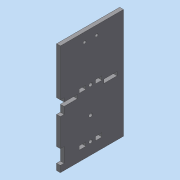
# Autodesk Inventor part: X-Motor-Housing_Side
Saved by Autodesk Inventor 2016 SP1 (Build 200210100, 210)
## iProperties
Created: 2016-02-23
Part Number: X-Motor-Housing_Side
Material: Generic
Document SubType Name: Modeling
Designer: Mohamed A.
Density: 1 g/cm^3
Appearance: Default
Author: Mohamed A.
Autodesk Inventor part; units mm, degrees
ref_plane "YZ Plane" through (0, 0, 0) normal (1, 0, 0) x (0, 1, 0)
ref_plane "XZ Plane" through (0, 0, 0) normal (0, 1, 0) x (-1, 0, 0)
ref_plane "XY Plane" through (0, 0, 0) normal (0, 0, 1) x (1, 0, 0)
sketch "Sketch2" plane through (0, 0, 0) normal (1, 0, 0) x (0, 1, 0)
  line L0 (-21, 22.5) -> (-21, 19.5)
  line L1 (-21, -11) -> (-21, -27.5)
  line L2 (-21, -27.5) -> (26, -27.5)
  line L3 (26, -27.5) -> (26, 27.5)
  line L4 (26, 27.5) -> (-21, 27.5)
  line L5 (-21, 27.5) -> (-21, 22.5)
  line L6 (26, 27.5) -> (26, 57.5)
  line L7 (26, 57.5) -> (-21, 57.5)
  line L8 (-21, 57.5) -> (-21, 27.5)
  circle A0 centre (4.7625, 50.5) radius 1.15
  circle A1 centre (-4.7625, 50.5) radius 1.15
  line L9 (4.7625, 50.5) -> (0, 50.5) construction
  line L10 (0, 50.5) -> (-4.7625, 50.5) construction
  line L11 (-21, 22.5) -> (-24, 22.5)
  line L12 (-24, 22.5) -> (-24, 57.5)
  line L13 (-24, 57.5) -> (-21, 57.5)
  line L14 (-21, -22.5) -> (-24, -22.5)
  line L15 (-24, -22.5) -> (-24, -27.5)
  line L16 (-24, -27.5) -> (-21, -27.5)
  line L17 (-21, -11) -> (-24, -11)
  line L18 (-24, -11) -> (-24, 11)
  line L19 (-24, 11) -> (-21, 11)
  line L20 (-21, 11) -> (-21, -11)
  line L21 (-21, 16.5) -> (-21, 11)
  line L22 (-21, 19.5) -> (-21, 16.5)
  circle A2 centre (0, 0) radius 1.4
  line L23 (10.5, 19.5) -> (21, 19.5) projected
  line L24 (10.5, 19.5) -> (10.5, 16.5) projected
  line L25 (21, 16.5) -> (10.5, 16.5) projected
  line L26 (21, 19.5) -> (21, 16.5) projected
  line L27 (3.75, 19.5) -> (9, 19.5) projected
  line L28 (9, 19.5) -> (9, 22.5) projected
  line L29 (3.75, 22.5) -> (9, 22.5) projected
  line L30 (3.75, 19.5) -> (3.75, 22.5) projected
  line L31 (-9, 19.5) -> (-3.75, 19.5) projected
  line L32 (-3.75, 19.5) -> (-3.75, 22.5) projected
  line L33 (-9, 22.5) -> (-3.75, 22.5) projected
  line L34 (-9, 19.5) -> (-9, 22.5) projected
  line L35 (-24, 19.5) -> (-10.5, 19.5) projected
  line L36 (-24, 19.5) -> (-24, 16.5) projected
  line L37 (-10.5, 16.5) -> (-24, 16.5) projected
  line L38 (-10.5, 19.5) -> (-10.5, 16.5) projected
  line L39 (0, -44.5) -> (0, 74.5) construction
  line L40 (-34, 0) -> (36, 0) construction
  line L41 (3.75, 22.5) -> (-3.75, 19.5) construction
  line L42 (3.75, 19.5) -> (-3.75, 22.5) construction
  circle A3 centre (0, 21) radius 1.4
  line L43 (-10.5, 16.5) -> (-21, 16.5)
  line L44 (-10.5, 16.5) -> (-10.5, 19.5)
  line L45 (-10.5, 19.5) -> (-21, 19.5)
  line L46 (-21, 16.5) -> (-21, 19.5)
  line L47 (9, -16.5) -> (3.75, -16.5) projected
  line L48 (3.75, -16.5) -> (3.75, -19.5) projected
  line L49 (9, -19.5) -> (3.75, -19.5) projected
  line L50 (9, -16.5) -> (9, -19.5) projected
  line L51 (-3.75, -16.5) -> (-9, -16.5) projected
  line L52 (-9, -16.5) -> (-9, -19.5) projected
  line L53 (-3.75, -19.5) -> (-9, -19.5) projected
  line L54 (-3.75, -16.5) -> (-3.75, -19.5) projected
  line L55 (3.75, -16.5) -> (-3.75, -19.5) construction
  line L56 (-3.75, -16.5) -> (3.75, -19.5) construction
  circle A4 centre (0, -18) radius 1.4
  dimension "d11" = 30
  dimension "d12" = 2.3
  dimension "d13" = 2.3
  dimension "d14" = 9.525
  dimension "d15" = 7
  dimension "d18" = 3
  dimension "d21" = 22
  dimension "d24" = 2.8
  dimension "d27" = 5
  dimension "d28" = 2.8
  dimension "d30" = 5
  dimension "d31" = 55
  dimension "d32" = 47
  dimension "d33" = 2.8
  constraints: 62 end point, 14 perpendicular, 10 collinear, 5 centre point, 5 horizontal, 3 point on line, 2 midpoint, 2 vertical, 1 coincident, 1 other
  measures "d11" distance of L3.end L6.end
  measures "d12" diameter of A0
  measures "d13" diameter of A1
  measures "d14" distance of L10.end L9.start
  measures "d15" distance between parallel lines of L9 L7
  measures "d18" distance of L1.start L17.end
  measures "d21" distance between parallel lines of L17 L19
  measures "d24" diameter of A2
  measures "d27" distance between parallel lines of L4 L33
  measures "d28" diameter of A3
  measures "d30" distance between parallel lines of L16 L14
  measures "d31" distance between parallel lines of L2 L4
  measures "d32" distance between parallel lines of L8 L6
  measures "d33" diameter of A4
extrude "Extrusion2" add sketch "Sketch2" along normal blind 3 contours L5 L4 L3 L2 L1 L20 L21 L37 L38 L35 L0 | L11 L12 L13 L8 L5 | L8 L7 L6 L4 | L20 L17 L18 L19 | L16 L15 L14 L1
body "Solid2"
